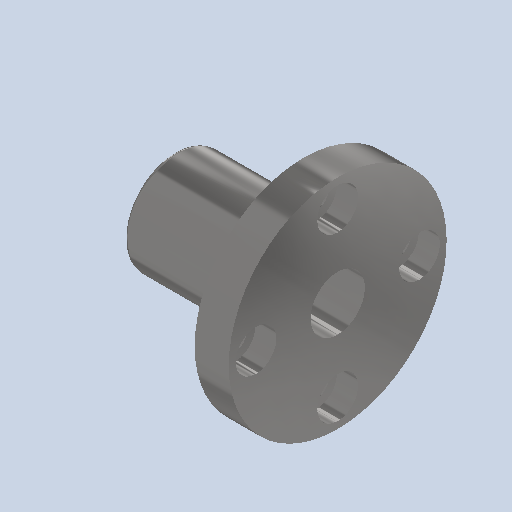
# Autodesk Inventor part: LHFR-N8
Saved by Autodesk Inventor 2022 (Build 260153000, 153)
## iProperties
Category: PARTsolutions
Company: MISUMI
Part Number: LHFR-N8
Material: 鉄、鋳鉄
Catalog Web Link: www.cadenas.de
Description: LHZR, LHFR-N, LHFR, LHFRF, LHFRR, LHFRM, LHFRMF, SLHFR, SLHFRS, LHZS, LHFS-N, LHFS, LHFSF, LHFSR, LHFSM, LHFSMF, SLHFS, SLHFSS,LHZC, LHFC-N, LHFC, LHFCF, LHFCR, LHFCM, LHFCMF, SLHFC, SLHFCS-Flanged Linear Bushings - Single Standard Type/Opposite Counterbore Hole Type
Vendor: MISUMI
Document SubType Name: Modeling
Designer: partserver
Manufacturer: MISUMI
Mass: 37 g
Surface Area: 37.599 cm^2
Volume: 5.72931 cm^3
Density: 6.45802 g/cm^3
Appearance: 鋼 - つや出し
PSOL_IDENT_0: {$CADENAS_DATA\23d-libs\misumi\metric\04_linear_bushings\lhfr_n.prj},369 {VTYP=3D},{NB=LHFR-N8},{LIN
PSOL_IDENT_1: A=LHFR-N8},{NN=LHZR, LHFR-N, LHFR, LHFRF, LHFRR, LHFRM, LHFRMF, SLHFR, SLHFRS, LHZS, LHFS-N, LHFS, L
PSOL_IDENT_2: HFSF, LHFSR, LHFSM, LHFSMF, SLHFS, SLHFSS,LHZC, LHFC-N, LHFC, LHFCF, LHFCR, LHFCM, LHFCMF, SLHFC, SL
PSOL_IDENT_3: HFCS},{DATE=30.10.2020 15:52:00},{GEOMDATE=27.08.2015 04:46:03},{VERSION=},{LINEID=50},{WBVAR=CH,TS,
PSOL_IDENT_4: TS1,MATOC,STOC,MATR,GREASE},{WBNUMERIC=}  {NB=LHFR-N8},{LINA=LHFR-N8},{KT=DUMMY},{PN=LHFR-N8},{CH=2}
PSOL_IDENT_5: ,{CHALG='1','Opposite Counterbore','2','Standard'},{TS=R},{TSAA= 'R','Round Flange', 'S','Square Fla
PSOL_IDENT_6: nge', 'C','2 - Flats Flange' },{TS1=-N},{TS1A= '-N','w/o Seal','','with Seal' },{MATOC=1},{MATOCAA= '
PSOL_IDENT_7: 1', '52100 Bearing Steel' },{HARDOC=58HRC~},{STOC=},{MATB=52100 Bearing Steel},{MATR=R},{MATRAA= 'R'
PSOL_IDENT_8: , 'Resin (Duracone M90 or Equivalent)' },{TYPE=LHFR},{OT=-20~80},{AC=Seal},{MATS=Nitrile Rubber (-20
PSOL_IDENT_9: ~120 deg Celsius)},{GREASE=},{DDRR=8},{DDRRTOL=0/-0.009},{D=15},{DTOL=0/-0.013},{L=24},{LTOL=±0.3},{
PSOL_IDENT_10: H=32},{T=5.0},{DD=3.5},{DD1=6.0},{TT=3.1},{PCD=24},{PCDFX=24},{W=0},{WFX=25},{F=0},{FFX=0},{A=0},{AF
PSOL_IDENT_11: X=24},{ESS=0.012},{PD=0.012},{BR=4},{CD=265},{CO=380},{MASS=37},{STAA= '','-' },{GREASEA='','N/A'},{
PSOL_IDENT_12: TIFF=1},{MATOCALG=},{STOCALG=},{MATRALG=}
NB: LHFR-N8
NN: LHZR, LHFR-N, LHFR, LHFRF, LHFRR, LHFRM, LHFRMF, SLHFR, SLHFRS, LHZS, LHFS-N, LHFS, LHFSF, LHFSR, LHFSM, LHFSMF, SLHFS, SLHFSS,LHZC, LHFC-N, LHFC, LHFCF, LHFCR, LHFCM, LHFCMF, SLHFC, SLHFCS
NT: Flanged Linear Bushings - Single Standard Type/Opposite Counterbore Hole Type
NBSYN: $PN.
LINA: LHFR-N8
CATALOG: Misumi
PN: LHFR-N8
CH: Standard
TS: Round Flange
TS1: w/o Seal
MATOC: 52100 Bearing Steel
HARDOC: 58HRC~
STOC: -
MATB: 52100 Bearing Steel
MATR: Resin (Duracone M90 or Equivalent)
OT: -20~80
AC: Seal
MATS: Nitrile Rubber (-20~120 deg Celsius)
GREASE: N/A
DDRR: 8
DDRRTOL: 0/-0.009
D: 15
DTOL: 0/-0.013
L: 24
LTOL: ±0.3
H: 32
T: 5
DD: 3.5
DD1: 6
TT: 3.1
PCD: 24
W: 0
F: 0
A: 0
ESS: 0.012
PD: 0.012
BR: 4
CD: 265
CO: 380
MASS: 37
SUPPLIER: MISUMI
ARTICLENO: LHFR-N8
BOMINFO: LHFR-N8
CREATOR: CADENAS GmbH
Title: LHFR-N8
Author: Cadenas PARTsolutions
Comments: Flanged Linear Bushings - Single Standard Type/Opposite Counterbore Hole Type
Autodesk Inventor part; units mm, degrees
sketch "Sketch_1" plane through (0, 0, 0) normal (0, 0, 1) x (1, 0, 0)
  line L0 (24, 0) -> (0, 0)
  line L1 (0, 4) -> (24, 4)
  line L2 (24, 4) -> (24, 6.75)
  arc A0 (24, 6.75) -> (23.25, 7.5) centre (23.25, 6.75) ccw
  line L3 (23.25, 7.5) -> (6, 7.5)
  line L4 (6, 7.5) -> (6, 7.2)
  line L5 (6, 7.2) -> (5, 7.2)
  line L6 (5, 7.2) -> (5, 16)
  line L7 (5, 16) -> (0, 16)
  line L8 (0, 16) -> (0, 4)
  constraints: 18 end point, 2 point on circle, 1 centre point
revolve "Revolution1" add sketch "Sketch_1" angle 360 about axis through (24, 0, 0) along (1, 0, 0)
sketch "Sketch2" plane through (0, 0, 0) normal (-1, 0, 0) x (0, 0, 1)
  point P0 (0, 12)
hole "Hole1" at (0, 12, 0) direction (1, 0, 0) diameter 3.5 depth 5 counterbore diameter 6 counterbore depth 3.1
sketch "Sketch3" plane through (0, 0, 0) normal (-1, 0, 0) x (0, 0, 1)
  point P0 (0, -12)
hole "Hole2" at (0, -12, 0) direction (1, 0, 0) diameter 3.5 depth 5 counterbore diameter 6 counterbore depth 3.1
sketch "Sketch4" plane through (0, 0, 0) normal (-1, 0, 0) x (0, 0, 1)
  point P0 (-12, 0)
hole "Hole3" at (0, 0, -12) direction (1, 0, 0) diameter 3.5 depth 5 counterbore diameter 6 counterbore depth 3.1
sketch "Sketch5" plane through (0, 0, 0) normal (-1, 0, 0) x (0, 0, 1)
  point P0 (12, 0)
hole "Hole4" at (0, 0, 12) direction (1, 0, 0) diameter 3.5 depth 5 counterbore diameter 6 counterbore depth 3.1
ref_plane "Combination_Module_XY" through (0, 0, 0) normal (1, 0, 0) x (0, 0, -1)
ref_plane "Combination_Module_YZ" through (0, 0, 0) normal (0, 0, -1) x (0, 1, 0)
ref_plane "Combination_Module_ZX" through (0, 0, 0) normal (0, 1, 0) x (1, 0, 0)
body "Solid1"
